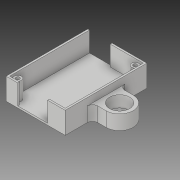
# Autodesk Inventor part: ResonanceBoardEnc
Saved by Autodesk Inventor 2019 (Build 230136000, 136)
## iProperties
Created: 2021-08-19
Part Number: ResonanceBoardEnc
Material: Generic
Document SubType Name: Modeling
Designer: devon
Density: 1 g/cm^3
Appearance: Default
Author: devon
Autodesk Inventor part; units mm, degrees
ref_plane "YZ Plane" through (0, 0, 0) normal (1, 0, 0) x (0, 1, 0)
ref_plane "XZ Plane" through (0, 0, 0) normal (0, 1, 0) x (-1, 0, 0)
ref_plane "XY Plane" through (0, 0, 0) normal (0, 0, 1) x (1, 0, 0)
sketch "Sketch1" plane through (0, 0, 0) normal (0, 1, 0) x (-1, 0, 0)
  line L0 (16.375, 22.625) -> (-16.375, 22.625)
  line L1 (-16.375, 22.625) -> (-16.375, -22.625)
  line L2 (-16.375, -22.625) -> (16.375, -22.625)
  line L3 (16.375, -22.625) -> (16.375, 22.625)
  line L4 (16.375, 22.625) -> (-16.375, -22.625) construction
  line L5 (-16.375, 22.625) -> (16.375, -22.625) construction
  point P0 (0, 0)
  dimension "d0" = 32.75
  dimension "d1" = 45.25
  constraints: 12 end point, 2 midpoint, 2 parallel, 1 horizontal, 1 perpendicular
  measures "d0" distance of L1.end L2.end
  measures "d1" distance of L0.end L1.end
extrude "Extrusion1" add sketch "Sketch1" along normal blind 12
sketch "Sketch2" plane through (0, 12, 0) normal (0, 1, 0) x (1, 0, 0)
  line L0 (-15.375, -21.625) -> (15.375, -21.625)
  line L1 (15.375, -21.625) -> (15.375, 21.625)
  line L2 (15.375, 21.625) -> (-15.375, 21.625)
  line L3 (-15.375, 21.625) -> (-15.375, -21.625)
  line L4 (-15.375, -21.625) -> (15.375, 21.625) construction
  line L5 (15.375, -21.625) -> (-15.375, 21.625) construction
  point P0 (0, 0)
  dimension "d4" = 30.75
  dimension "d5" = 43.25
  constraints: 12 end point, 2 midpoint, 2 parallel, 1 horizontal, 1 perpendicular
  measures "d4" distance of L1.end L2.end
  measures "d5" distance of L0.end L1.end
extrude "Extrusion2" cut sketch "Sketch2" against normal blind 11
sketch "Sketch5" plane through (0, 1, 0) normal (0, 1, 0) x (1, 0, 0)
  circle A0 centre (13.125, 19.375) radius 2
  circle A1 centre (-13.125, -19.375) radius 2
  line L0 (15.375, 21.625) -> (15.375, -21.625) projected
  line L1 (-15.375, 21.625) -> (15.375, 21.625) projected
  line L2 (-15.375, -21.625) -> (-15.375, 21.625) projected
  line L3 (15.375, -21.625) -> (-15.375, -21.625) projected
  point P0 (0, 0)
  dimension "d20" = 4
  dimension "d21" = 2.25
  dimension "d22" = 2.25
  dimension "d23" = 2.25
  dimension "d24" = 2.25
  dimension "d25" = 4
  constraints: 2 centre point
  measures "d20" diameter of A0
  measures "d21" distance from line of L0 A0.centre
  measures "d22" distance from line of L1 A0.centre
  measures "d23" distance from line of L2 A1.centre
  measures "d24" distance from line of L3 A1.centre
  measures "d25" diameter of A1
extrude "Extrusion5" add sketch "Sketch5" along normal blind 10 contours A0 | A1
sketch "Sketch6" plane through (13.125, 11, -19.375) normal (0, 1, 0) x (1, 0, 0)
  circle A0 centre (-26.25, -38.75) radius 2 projected
  circle A1 centre (-26.25, -38.75) radius 1
  circle A2 centre (0, 0) radius 2 projected
  circle A3 centre (0, 0) radius 1
  point P0 (-13.125, -19.375)
  dimension "d28" = 2
  dimension "d29" = 2
  constraints: 2 centre point, 2 coincident
  measures "d28" diameter of A1
  measures "d29" diameter of A3
extrude "Extrusion6" cut sketch "Sketch6" against normal blind 10 contours A1 | A3
sketch "Sketch7" plane through (0, 12, 0) normal (0, 1, 0) x (1, 0, 0)
  line L0 (16.375, 22.625) -> (-16.375, 22.625) projected
  line L1 (-15.375, 21.625) -> (-2.875, 21.625)
  line L2 (-2.875, 21.625) -> (-2.875, 22.625)
  line L3 (-2.875, 22.625) -> (-15.375, 22.625)
  line L4 (-15.375, 22.625) -> (-15.375, 21.625)
  line L5 (15.375, -21.625) -> (-15.375, -21.625) projected
  line L6 (-16.375, -22.625) -> (16.375, -22.625) projected
  line L7 (-9.875, -21.625) -> (6.625, -21.625)
  line L8 (6.625, -21.625) -> (6.625, -22.625)
  line L9 (6.625, -22.625) -> (-9.875, -22.625)
  line L10 (-9.875, -22.625) -> (-9.875, -21.625)
  line L11 (-15.375, -21.625) -> (-15.375, 21.625) projected
  point P0 (0, 0)
  dimension "d32" = 12.5
  dimension "d33" = 5.5
  dimension "d35" = 22
  constraints: 16 end point, 4 parallel, 3 point on line, 2 horizontal, 2 perpendicular
  measures "d32" distance between parallel lines of L2 L4
  measures "d33" distance between parallel lines of L11 L10
  measures "d35" distance between parallel lines of L11 L8
extrude "Extrusion7" cut sketch "Sketch7" against normal blind 11
sketch "Sketch8" plane through (0, 0, 0) normal (0, -1, 0) x (1, 0, 0)
  line L0 (16.375, 22.625) -> (16.375, -22.625) projected
  line L1 (16.375, 7.5) -> (31.375, 7.5)
  line L2 (31.375, 7.5) -> (31.375, -7.5)
  line L3 (31.375, -7.5) -> (16.375, -7.5)
  line L4 (16.375, -7.5) -> (16.375, 7.5)
  point P0 (0, 0)
  dimension "d38" = 15
  dimension "d39" = 7.5
  dimension "d40" = 15
  constraints: 8 end point, 2 parallel, 1 horizontal, 1 perpendicular, 1 point on line
  measures "d38" distance of L1.end L2.end
  measures "d39" distance from line of point (0, 0) L3
  measures "d40" distance of L1.start L1.end
extrude "Extrusion8" add sketch "Sketch8" against normal blind 8
sketch "Sketch9" plane through (0, 8, 0) normal (0, 1, 0) x (1, 0, 0)
  line L0 (31.375, -7.5) -> (31.375, 7.5) projected
  point P0 (0, 0)
  point P1 (23.875, 0.0223)
  dimension "d50" = 7.5
  measures "d50" distance from line of L0 point (23.875, 0.022)
hole "Hole1" at (23.875, 8, -0.0223) direction (0, -1, 0) diameter 6.756 depth 10.9728 tip angle 118 counterbore diameter 11.113 counterbore depth 6.35 clearance for "Socket Head Cap Screw" size "1/4" standard "Ansi Unified Screw Threads"
fillet "Fillet1" radius 3 2 edges at (16.375, 4, -7.5) (16.375, 4, 7.5)
fillet "Fillet2" radius 7.5 2 edges at (31.375, 4, -7.5) (31.375, 4, 7.5)
body "Solid1"
